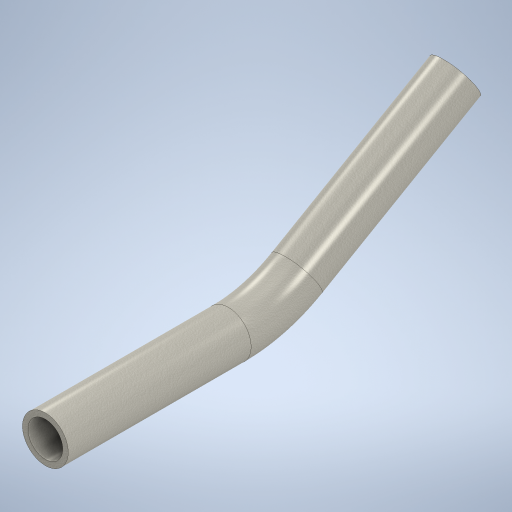
# Autodesk Inventor part: TB11GA1330
Saved by Autodesk Inventor 2023 (Build 270158000, 158)
## iProperties
RuleStatus: InUse
Created: 2023-02-03
Part Number: TB11GA1330
Material: Generic
Document SubType Name: Modeling
Designer: Admin
Density: 1 g/cm^3
Appearance: Steel - Cast
Author: Admin
Autodesk Inventor part; units mm, degrees
ref_plane "YZ Plane" through (0, 0, 0) normal (1, 0, 0) x (0, 1, 0)
ref_plane "XZ Plane" through (0, 0, 0) normal (0, 1, 0) x (-1, 0, 0)
ref_plane "XY Plane" through (0, 0, 0) normal (0, 0, 1) x (1, 0, 0)
sketch "Sketch1" plane through (0, 0, 0) normal (1, 0, 0) x (0, 1, 0)
  line L0 (0, 0) -> (0, -101.6)
  arc A0 (0, -101.6) -> (10.2089, -139.7) centre (76.2, -101.6) ccw
  line L1 (10.2089, -139.7) -> (61.0089, -227.6882)
  dimension "bendAngleSketch" = 150
  dimension "CLR" = 76.2
  dimension "ST" = 101.6
  constraints: 4 end point, 2 point on circle, 2 tangent, 1 centre point, 1 equal length, 1 vertical
  measures "bendAngleSketch" angle of L1 L0
  measures "CLR" radius of A0
  measures "ST" distance of L0.start L0.end
sketch "Sketch2" plane through (0, 0, 0) normal (0, 0, 1) x (1, 0, 0)
  circle A0 centre (0, 0) radius 12.7
  circle A1 centre (0, 0) radius 9.652
  dimension "outerDiameter" = 25.4
  dimension "wallThickness" = 3.048
  constraints: 2 centre point, 1 coincident
  measures "outerDiameter" diameter of A0
  measures "wallThickness" radial gap between concentric circles of A0 A1
sweep "Sweep1" add profiles "Sketch2" path "Sketch1"
equation "\"bendAngle\" = 30deg"
body "Solid1"
